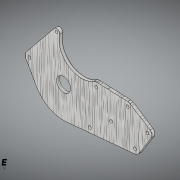
# Autodesk Inventor part: 後ろ脚内内フレーム
Saved by Autodesk Inventor 2019 (Build 230136000, 136)
## iProperties
Created: 2019-11-28
Part Number: 後ろ脚内内フレーム
Material: アルミニウム 7075
Document SubType Name: Modeling
Designer: tanjihayato
Density: 2.81 g/cm^3
Appearance: サテン - ブラシ仕上げ 重厚
Author: tanjihayato
Autodesk Inventor part; units mm, degrees
ref_plane "YZ Plane" through (0, 0, 0) normal (1, 0, 0) x (0, 1, 0)
ref_plane "XZ Plane" through (0, 0, 0) normal (0, 1, 0) x (-1, 0, 0)
ref_plane "XY Plane" through (0, 0, 0) normal (0, 0, 1) x (1, 0, 0)
sketch "スケッチ1" plane through (0, 0, 0) normal (0, 0, 1) x (1, 0, 0)
  circle A0 centre (-21.6908, -16.4118) radius 1.5
  circle A1 centre (-58.0056, -24.4791) radius 1.5
  circle A2 centre (-34.2292, -36.4056) radius 1.5
  circle A3 centre (-41.5152, -3.6073) radius 1.5
  circle A4 centre (-72.8083, -2.3784) radius 1.5
  circle A5 centre (-79.2726, -40.4563) radius 1.5
  line L0 (-149.4523, -1.6098) -> (-132.6633, -31.6026) construction
  circle A6 centre (-105.5257, -16.4118) radius 30.1 construction
  arc A7 (-143.0373, -7.2595) -> (-143.4712, -12.2949) centre (-139.5445, -10.0968) ccw
  circle A8 centre (-139.5445, -10.0968) radius 1.5
  circle A9 centre (-105.5257, -16.4118) radius 7.025
  line L1 (-21.6908, -16.4118) -> (-91.5316, 55.2499) construction
  line L2 (-21.6908, -16.4118) -> (-120.9187, -3.4901) construction
  line L3 (-91.5316, 55.2499) -> (-49.8446, 17.1127) construction
  line L4 (-49.8446, 17.1127) -> (-120.9187, -3.4901) construction
  line L5 (-105.5257, -16.4118) -> (-21.6908, -16.4118) construction
  line L6 (-21.6908, -16.4118) -> (-99.9742, 13.5882) construction
  line L7 (-21.6908, -16.4118) -> (-101.7113, -41.4118) construction
  line L8 (-21.6908, -16.4118) -> (-112.5507, 25.5122) construction
  line L9 (-112.5507, 25.5122) -> (-49.8446, 17.1127) construction
  circle A10 centre (-112.5507, 25.5122) radius 1.25
  arc A11 (-109.6144, 24.8971) -> (-114.8792, 27.4038) centre (-112.5507, 25.5122) ccw
  arc A12 (-17.8785, -18.8026) -> (-19.2493, -12.6317) centre (-21.6908, -16.4118) ccw
  circle A13 centre (-58.0056, -24.4791) radius 4.5 construction
  arc A14 (-33.8066, -40.8857) -> (-30.4168, -38.7963) centre (-34.2292, -36.4056) ccw
  circle A15 centre (-79.2726, -40.4563) radius 4.5 construction
  arc A16 (-39.0737, 0.1727) -> (-41.3386, 0.8892) centre (-41.5152, -3.6073) ccw
  arc A17 (-72.6317, 2.1181) -> (-75.2637, 1.3927) centre (-72.8083, -2.3784) ccw
  arc A18 (-132.6633, -31.6026) -> (-102.6055, -47.3744) centre (-105.5257, -16.4118) ccw
  line L10 (-33.8066, -40.8857) -> (-102.6055, -47.3744)
  line L11 (-30.4168, -38.7963) -> (-17.8785, -18.8026)
  line L12 (-19.2493, -12.6317) -> (-39.0737, 0.1727)
  line L13 (-72.6317, 2.1181) -> (-41.3386, 0.8892)
  arc A19 (-109.6144, 24.8971) -> (-75.2637, 1.3927) centre (-87.5593, 20.2765) ccw
  line L14 (-143.4712, -12.2949) -> (-132.6633, -31.6026)
  line L15 (-143.0373, -7.2595) -> (-114.8792, 27.4038)
  point P0 (0, 0)
  point P1 (0, 0)
  point P2 (0, 0)
  dimension "d16" = 9
  dimension "d17" = 3
  dimension "d18" = 56.5
  dimension "d19" = 74
  dimension "d20" = 17.35
  dimension "d21" = 20.968
  dimension "d22" = 17.35
  dimension "d23" = 20.968
  dimension "d24" = 2.5
  dimension "d25" = 3
  dimension "d26" = 3
  dimension "d27" = 3
  dimension "d28" = 3
  dimension "d29" = 3
  dimension "d30" = 3
  dimension "d31" = 3
  constraints: 32 end point, 20 centre point, 17 point on circle, 16 tangent, 3 coincident, 2 equal length
  measures "d16" diameter of A7
  measures "d17" diameter of A8
  measures "d18" distance of L1.end L3.end
  measures "d19" distance of L3.end L2.end
  measures "d20" angle of L5 L7
  measures "d21" angle of L6 L5
  measures "d22" angle of L8 L2
  measures "d23" angle of L8 L1
  measures "d24" diameter of A10
  measures "d25" radial gap between concentric circles of A0 A12
  measures "d26" radial gap between concentric circles of A1 A13
  measures "d27" radial gap between concentric circles of A2 A14
  measures "d28" radial gap between concentric circles of A5 A15
  measures "d29" radial gap between concentric circles of A3 A16
  measures "d30" radial gap between concentric circles of A4 A17
  measures "d31" radius of A11
extrude "押し出し1" add sketch "スケッチ1" along normal blind 3
equation "\"d22\" = d20"
equation "\"d23\" = d21"
